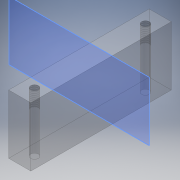
# Autodesk Inventor part: ImagineFrameSides
Saved by Autodesk Inventor 2018 (Build 220112000, 112)
## iProperties
Created: 2020-09-26
Part Number: ImagineFrameSides
Material: SAN Plastic
Document SubType Name: Modeling
Designer: Lveli
Density: 1.068 g/cm^3
Appearance: Polycarbonate - Clear
Author: Lveli
Autodesk Inventor part; units mm, degrees
ref_plane "YZ Plane" through (0, 0, 0) normal (1, 0, 0) x (0, 1, 0)
ref_plane "XZ Plane" through (0, 0, 0) normal (0, 1, 0) x (-1, 0, 0)
ref_plane "XY Plane" through (0, 0, 0) normal (0, 0, 1) x (1, 0, 0)
sketch "Sketch1" plane through (0, 0, 0) normal (0, 0, 1) x (1, 0, 0)
  line L0 (0, 0) -> (9.525, 0)
  line L1 (9.525, 0) -> (9.525, 25.4)
  line L2 (9.525, 25.4) -> (0, 25.4)
  line L3 (0, 25.4) -> (0, 0)
  dimension "d0" = 9.525
  dimension "d1" = 25.4
  constraints: 8 end point, 2 parallel, 1 horizontal, 1 perpendicular
  measures "d0" distance of L2.end L1.end
  measures "d1" distance of L1.end L0.end
extrude "Extrusion1" add sketch "Sketch1" along normal blind 60.325
sketch "Sketch2" plane through (0, 25.4, 0) normal (0, 1, 0) x (1, 0, 0)
  line L0 (0, 0) -> (0, -60.325) construction
  line L1 (9.525, -60.325) -> (0, -60.325) construction
  line L2 (0, -30.1625) -> (9.525, -30.1625) construction
  point P0 (4.7625, -53.975)
  point P1 (4.7625, -6.35)
  dimension "d4" = 4.7625
  dimension "d5" = 6.35
  constraints: 2 end point, 1 horizontal, 1 midpoint, 1 symmetric about line
  measures "d4" distance from line of L0 point (4.763, -53.975)
  measures "d5" distance from line of L1 point (4.763, -53.975)
hole "Hole1" at (4.7625, 25.4, 53.975) at (4.7625, 25.4, 6.35) direction (0, -1, 0) diameter 3.302 end through all thread size "8-32 UNC" class "2B" standard "ANSI Unified Screw Threads"
body "Solid1"
